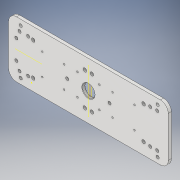
# Autodesk Inventor part: Base Plate New
Saved by Autodesk Inventor 2019 (Build 230136000, 136)
## iProperties
Created: 2019-10-06
Part Number: Base Plate New
Material: UHMW, White
Document SubType Name: Modeling
Designer: robgr
Density: 0.94 g/cm^3
Appearance: Smooth - White
Mass: 52.7671 g
Surface Area: 319.531 cm^2
Volume: 56.1352 cm^3
Author: robgr
Autodesk Inventor part; units mm, degrees
(part 1 of 2)
ref_plane "YZ Plane" through (0, 0, 0) normal (1, 0, 0) x (0, 1, 0)
sketch "Sketch1" plane through (0, 0, 0) normal (0, 0, 1) x (1, 0, 0)
  line L0 (-19.3782, 63.0791) -> (164.6218, 63.0791)
  line L1 (174.6218, 53.0791) -> (174.6218, 1.0791)
  line L2 (164.6218, -8.9209) -> (-19.3782, -8.9209)
  line L3 (-29.3782, 1.0791) -> (-29.3782, 53.0791)
  arc A0 (-19.3782, 63.0791) -> (-29.3782, 53.0791) centre (-19.3782, 53.0791) ccw
  arc A1 (-29.3782, 1.0791) -> (-19.3782, -8.9209) centre (-19.3782, 1.0791) ccw
  arc A2 (164.6218, -8.9209) -> (174.6218, 1.0791) centre (164.6218, 1.0791) ccw
  arc A3 (174.6218, 53.0791) -> (164.6218, 63.0791) centre (164.6218, 53.0791) ccw
  point P0 (0, 0)
  point P1 (-29.3782, 63.0791)
  point P2 (174.6218, -8.9209)
  point P3 (-29.3782, -8.9209)
  dimension "d0" = 204
  dimension "d1" = 72
  dimension "d2" = 10
  constraints: 8 end point, 8 point on circle, 8 tangent, 6 point on line, 4 centre point, 3 equal radius, 2 parallel, 1 horizontal, 1 perpendicular
  measures "d0" distance of point (174.622, -8.921) point (-29.378, -8.921)
  measures "d1" distance of point (-29.378, -8.921) point (-29.378, 63.079)
  measures "d2" radius of A0
extrude "Extrusion1" add sketch "Sketch1" along normal blind 4
sketch "Sketch3" plane through (0, 0, 0) normal (0, 0, -1) x (-1, 0, 0)
  circle A0 centre (19.3782, 39.5791) radius 2
  line L0 (29.3782, 1.0791) -> (29.3782, 53.0791) projected
  circle A1 centre (19.3782, 14.5791) radius 2
  circle A2 centre (19.3782, 53.0791) radius 2 projected
  circle A3 centre (19.3782, 1.0791) radius 2 projected
  line L1 (29.3782, 53.0791) -> (29.3782, 1.0791) projected
  line L2 (29.3782, 27.0791) -> (-174.6218, 27.0791)
  line L3 (-174.6218, 1.0791) -> (-174.6218, 53.0791) projected
  point P0 (0, 0)
  dimension "d10" = 4
  dimension "d15" = 25
  dimension "d16" = 12.5
  constraints: 2 centre point, 2 end point, 2 midpoint
  measures "d10" diameter of A0
  measures "d15" distance of A1.centre A0.centre
  measures "d16" distance from line of L2 A0.centre
extrude "Extrusion3" cut sketch "Sketch3" against normal blind 6 contours A0 | A1
sketch "Sketch4" plane through (0, 0, 4) normal (0, 0, 1) x (1, 0, 0)
  circle A0 centre (-4.3782, 5.0791) radius 2
  circle A1 centre (-19.3782, 14.5791) radius 2 projected
  circle A2 centre (-4.3782, 49.0791) radius 2
  circle A3 centre (-19.3782, 39.5791) radius 2 projected
  line L0 (164.6218, 63.0791) -> (-19.3782, 63.0791) projected
  line L1 (72.6218, 63.0791) -> (72.6218, -8.9209)
  line L2 (-19.3782, -8.9209) -> (164.6218, -8.9209) projected
  circle A4 centre (151.6218, 5.0791) radius 2
  circle A5 centre (151.6218, 49.0791) radius 2
  line L3 (174.6218, 1.0791) -> (174.6218, 53.0791) projected
  line L4 (-29.3782, 53.0791) -> (-29.3782, 1.0791) projected
  point P0 (0, 0)
  dimension "d17" = 4
  dimension "d19" = 4
  dimension "d37" = 23
  dimension "d38" = 14
  dimension "d39" = 14
  dimension "d40" = 23
  dimension "d41" = 25
  dimension "d42" = 14
  dimension "d43" = 25
  dimension "d44" = 14
  constraints: 4 centre point, 2 end point, 2 midpoint
  measures "d17" diameter of A0
  measures "d19" diameter of A2
  measures "d37" distance from line of L3 A4.centre
  measures "d38" distance from line of L2 A4.centre
  measures "d39" distance from line of L0 A5.centre
  measures "d40" distance from line of L3 A5.centre
  measures "d41" distance from line of L4 A2.centre
  measures "d42" distance from line of L0 A2.centre
  measures "d43" distance from line of L4 A0.centre
  measures "d44" distance from line of L2 A0.centre
extrude "Extrusion4" cut sketch "Sketch4" against normal blind 60 contours A0 | A2 | A4 | A5
ref_plane "Work Plane1" through (74.6218, 1.0791, 0) normal (1, 0, 0) x (0, 0, -1)
ref_plane "Work Plane2" through (-19.3782, 27.0791, 0) normal (0, -1, 0) x (1, 0, 0)
ref_plane "Work Plane3" through (-19.3782, 27.0791, 4) normal (0, 1, 0) x (1, 0, 0)
sketch "Sketch7" plane through (0, 0, 4) normal (0, 0, 1) x (1, 0, 0)
  point P0 (0, 0)
sketch "Sketch8" plane through (0, 0, 4) normal (0, 0, 1) x (1, 0, 0)
  circle A0 centre (-13.8782, -1.9209) radius 2
  line L0 (-19.3782, -8.9209) -> (164.6218, -8.9209) projected
  line L1 (-29.3782, 53.0791) -> (-29.3782, 1.0791) projected
  circle A1 centre (-13.8782, 56.0791) radius 2
  line L2 (164.6218, 63.0791) -> (-19.3782, 63.0791) projected
  circle A2 centre (161.1218, 56.0791) radius 2
  line L3 (174.6218, 1.0791) -> (174.6218, 53.0791) projected
  circle A3 centre (161.1218, -1.9209) radius 2
  point P0 (0, 0)
  dimension "d45" = 4
  dimension "d46" = 7
  dimension "d47" = 15.5
  dimension "d48" = 4
  dimension "d49" = 7
  dimension "d50" = 15.5
  dimension "d51" = 4
  dimension "d52" = 7
  dimension "d53" = 13.5
  constraints: 4 centre point
  measures "d45" diameter of A0
  measures "d46" distance from line of L0 A0.centre
  measures "d47" distance from line of L1 A0.centre
  measures "d48" diameter of A1
  measures "d49" distance from line of L2 A1.centre
  measures "d50" distance from line of L1 A1.centre
  measures "d51" diameter of A2
  measures "d52" distance from line of L2 A2.centre
  measures "d53" distance from line of L3 A2.centre
extrude "Extrusion6" cut sketch "Sketch8" against normal blind 10
sketch "Sketch9" plane through (0, 0, 4) normal (0, 0, 1) x (1, 0, 0)
  line L0 (-29.3782, 53.0791) -> (-29.3782, 1.0791) projected
  line L1 (-29.3782, 27.0791) -> (174.6218, 27.0791)
  line L2 (174.6218, 53.0791) -> (174.6218, 1.0791) projected
  line L3 (164.6218, 63.0791) -> (-19.3782, 63.0791) projected
  line L4 (72.6218, 63.0791) -> (72.6218, -8.9209)
  line L5 (164.6218, -8.9209) -> (-19.3782, -8.9209) projected
  circle A0 centre (72.6218, 27.0791) radius 8
  circle A1 centre (13.7163, 41.0791) radius 1
  circle A2 centre (41.7163, 41.0791) radius 1.0089
  circle A3 centre (41.7163, 13.0791) radius 1
  circle A4 centre (13.7163, 13.0791) radius 1
  circle A5 centre (77.0888, 48.0791) radius 2.225
  circle A6 centre (143.1888, 48.0791) radius 2.225
  circle A7 centre (143.1888, 6.0791) radius 2.225
  circle A8 centre (77.0888, 6.0791) radius 2.225
  point P0 (0, 0)
  dimension "d56" = 16
  dimension "d57" = 2
  dimension "d58" = 2
  dimension "d59" = 28
  dimension "d60" = 28
  dimension "d61" = 28
  dimension "d62" = 28
  dimension "d63" = 22
  dimension "d64" = 4.45
  dimension "d65" = 66.1
  dimension "d66" = 4.45
  dimension "d67" = 42
  dimension "d68" = 42
  dimension "d69" = 66.1
  dimension "d70" = 15
  dimension "d71" = 15
  dimension "d73" = 22
  constraints: 9 centre point, 5 midpoint, 4 end point
  measures "d56" diameter of A0
  measures "d57" diameter of A1
  measures "d58" diameter of A3
  measures "d59" distance of A2.centre A1.centre
  measures "d60" distance of A4.centre A1.centre
  measures "d61" distance of A3.centre A4.centre
  measures "d62" distance of A2.centre A3.centre
  measures "d63" distance from line of L3 A1.centre
  measures "d64" diameter of A5
  measures "d65" distance of A5.centre A6.centre
  measures "d66" diameter of A7
  measures "d67" distance of A7.centre A6.centre
  measures "d68" distance of A8.centre A5.centre
  measures "d69" distance of A7.centre A8.centre
  measures "d70" distance from line of L3 A5.centre
  measures "d71" distance from line of L5 A8.centre
  measures "d73" distance from line of L5 A4.centre
extrude "Extrusion7" cut sketch "Sketch9" against normal blind 10
ref_plane "Work Plane4" through (72.6218, 1.0791, 0) normal (1, 0, 0) x (0, 0, -1)
mirror "Mirror2" about plane through (72.6218, 1.0791, 0) normal (1, 0, 0) of "Extrusion7"
sketch "Sketch10" plane through (0, 0, 4) normal (0, 0, 1) x (1, 0, 0)
  line L0 (164.6218, 63.0791) -> (-19.3782, 63.0791) projected
  line L1 (72.6218, 63.0791) -> (72.6218, -8.9209)
  line L2 (-19.3782, -8.9209) -> (164.6218, -8.9209) projected
  line L3 (-29.3782, 53.0791) -> (-29.3782, 1.0791) projected
  line L4 (-29.3782, 27.0791) -> (174.6218, 27.0791)
  line L5 (174.6218, 1.0791) -> (174.6218, 53.0791) projected
  circle A0 centre (-15.3782, 49.0791) radius 2
  circle A1 centre (160.6218, 49.0791) radius 2
  circle A2 centre (-15.3782, 5.0791) radius 2
  circle A3 centre (160.6218, 5.0791) radius 2
  point P0 (0, 0)
  dimension "d77" = 4
  dimension "d78" = 14
  dimension "d79" = 14
  constraints: 4 centre point, 4 end point, 4 midpoint, 3 symmetric about line, 3 other
  measures "d77" diameter of A0
  measures "d78" distance from line of L0 A0.centre
  measures "d79" distance from line of L3 A0.centre
extrude "Extrusion8" cut sketch "Sketch10" against normal blind 10
sketch "Sketch11" plane through (0, 0, 4) normal (0, 0, 1) x (1, 0, 0)
  circle A0 centre (58.6218, 13.0791) radius 1.1
  circle A1 centre (58.6218, 41.0791) radius 1.1
  circle A2 centre (86.6218, 41.0791) radius 1.1
  circle A3 centre (86.6218, 13.0791) radius 1.1
  circle A4 centre (72.6218, 27.0791) radius 8 projected
  point P0 (0, 0)
  dimension "d82" = 2.2
  dimension "d83" = 2.2
  dimension "d84" = 2.2
  dimension "d85" = 28
  dimension "d86" = 28
  dimension "d87" = 28
  dimension "d88" = 28
  dimension "d89" = 14
  dimension "d90" = 14
  dimension "d91" = 14
  dimension "d92" = 14
  constraints: 4 centre point
  measures "d82" diameter of A0
  measures "d83" diameter of A1
  measures "d84" diameter of A2
  measures "d85" distance of A2.centre A1.centre
  measures "d86" distance of A1.centre A0.centre
  measures "d87" distance of A3.centre A0.centre
  measures "d88" distance of A2.centre A3.centre
  measures "d89" horizontal distance of A0.centre A4.centre
  measures "d90" horizontal distance of A3.centre A4.centre
  measures "d91" horizontal distance of A2.centre A4.centre
  measures "d92" horizontal distance of A4.centre A1.centre
extrude "Extrusion9" cut sketch "Sketch11" against normal blind 10 contours A0 | A1 | A2 | A3
fillet "Fillet1" radius 0.5 2 edges at (64.6218, 27.0791, 4) (64.6218, 27.0791, 0)
sketch "Sketch12" plane through (0, 0, 4) normal (0, 0, 1) x (1, 0, 0)
  line L0 (-29.3782, 1.0791) -> (-29.3782, 53.0791) projected
  line L1 (-29.3782, 27.0791) -> (174.6218, 27.0791)
  line L2 (174.6218, 53.0791) -> (174.6218, 1.0791) projected
  circle A0 centre (45.6218, 27.0791) radius 2
  circle A1 centre (99.6218, 27.0791) radius 2
  point P0 (0, 0)
  dimension "d96" = 4
  dimension "d97" = 4
  dimension "d98" = 75
  dimension "d99" = 75
  constraints: 2 centre point, 2 end point, 2 midpoint, 2 point on line
  measures "d96" diameter of A0
  measures "d97" diameter of A1
  measures "d98" distance from line of L0 A0.centre
  measures "d99" distance from line of L2 A1.centre
extrude "Extrusion10" cut sketch "Sketch12" against normal blind 10
sketch "Sketch13" plane through (0, 0, 0) normal (0, 0, -1) x (-1, 0, 0)
  line L0 (-128.4589, -1.8253) -> (-20.3883, -1.8253) construction
  line L1 (-20.3883, -1.8253) -> (-20.3883, -5.9209) construction
  line L2 (-20.3883, -5.9209) -> (-128.4589, -5.9209) construction
  line L3 (-128.4589, -5.9209) -> (-128.4589, -1.8253) construction
  line L4 (-164.6218, -8.9209) -> (19.3782, -8.9209) projected
  line L5 (-60.6379, 54.6498) -> (-88.5532, 54.6498) construction
  line L6 (-88.5532, 54.6498) -> (-88.5532, 60.0791) construction
  line L7 (-88.5532, 60.0791) -> (-60.6379, 60.0791) construction
  line L8 (-60.6379, 60.0791) -> (-60.6379, 54.6498) construction
  line L9 (19.3782, 63.0791) -> (-164.6218, 63.0791) projected
  line L10 (-125.7913, -5.029) -> (-126.3174, -5.029)
  line L11 (-126.3174, -5.029) -> (-127.2807, -3.8162)
  line L12 (-127.2807, -3.8162) -> (-127.7451, -3.8162)
  line L13 (-127.7451, -3.8162) -> (-127.7451, -5.029)
  line L14 (-127.7451, -5.029) -> (-128.1501, -5.029)
  line L15 (-128.1501, -5.029) -> (-128.1501, -1.981)
  line L16 (-128.1501, -1.981) -> (-127.3647, -1.981)
  spline S0 degree 2 poles (-127.3647, -1.981) (-127.1029, -1.981) (-126.7496, -2.0378) (-126.5891, -2.1415) knots 0 0 0 1 2 2 2
  spline S1 degree 2 poles (-126.5891, -2.1415) (-126.4285, -2.2452) (-126.2433, -2.5688) (-126.2433, -2.8084) knots 0 0 0 1 2 2 2
  spline S2 degree 2 poles (-126.2433, -2.8084) (-126.2433, -3.1419) (-126.5841, -3.5939) (-126.8756, -3.7026) knots 0 0 0 1 2 2 2
  line L17 (-126.8756, -3.7026) -> (-125.7913, -5.029)
  spline S3 degree 2 poles (-126.6657, -2.8405) (-126.6657, -2.7071) (-126.7595, -2.5021) (-126.8583, -2.4354) knots 0 0 0 1 2 2 2
  spline S4 degree 2 poles (-126.8583, -2.4354) (-126.9448, -2.3786) (-127.1745, -2.3317) (-127.3424, -2.3317) knots 0 0 0 1 2 2 2
  line L18 (-127.3424, -2.3317) -> (-127.7451, -2.3317)
  line L19 (-127.7451, -2.3317) -> (-127.7451, -3.4778)
  line L20 (-127.7451, -3.4778) -> (-127.3894, -3.4778)
  spline S5 degree 2 poles (-127.3894, -3.4778) (-127.214, -3.4778) (-126.9349, -3.416) (-126.8386, -3.3197) knots 0 0 0 1 2 2 2
  spline S6 degree 2 poles (-126.8386, -3.3197) (-126.7496, -3.2357) (-126.6657, -2.9986) (-126.6657, -2.8405) knots 0 0 0 1 2 2 2
  spline S7 degree 2 poles (-123.6992, -3.8853) (-123.6992, -4.4633) (-124.2549, -5.0932) (-124.7193, -5.0932) knots 0 0 0 1 2 2 2
  spline S8 degree 2 poles (-124.7193, -5.0932) (-125.196, -5.0932) (-125.7419, -4.4436) (-125.7419, -3.8853) knots 0 0 0 1 2 2 2
  spline S9 degree 2 poles (-125.7419, -3.8853) (-125.7419, -3.3123) (-125.1787, -2.6775) (-124.7193, -2.6775) knots 0 0 0 1 2 2 2
  spline S10 degree 2 poles (-124.7193, -2.6775) (-124.2549, -2.6775) (-123.6992, -3.3098) (-123.6992, -3.8853) knots 0 0 0 1 2 2 2
  spline S11 degree 2 poles (-124.0968, -3.8853) (-124.0968, -3.4407) (-124.4204, -3.0085) (-124.7193, -3.0085) knots 0 0 0 1 2 2 2
  spline S12 degree 2 poles (-124.7193, -3.0085) (-125.0182, -3.0085) (-125.3442, -3.4407) (-125.3442, -3.8853) knots 0 0 0 1 2 2 2
  spline S13 degree 2 poles (-125.3442, -3.8853) (-125.3442, -4.3176) (-125.0182, -4.7622) (-124.7193, -4.7622) knots 0 0 0 1 2 2 2
  spline S14 degree 2 poles (-124.7193, -4.7622) (-124.4229, -4.7622) (-124.0968, -4.325) (-124.0968, -3.8853) knots 0 0 0 1 2 2 2
  spline S15 degree 2 poles (-121.3872, -3.8483) (-121.3872, -4.409) (-121.9306, -5.0932) (-122.3407, -5.0932) knots 0 0 0 1 2 2 2
  spline S16 degree 2 poles (-122.3407, -5.0932) (-122.5259, -5.0932) (-122.7902, -5.0018) (-122.9186, -4.9227) knots 0 0 0 1 2 2 2
  line L21 (-122.9186, -4.9227) -> (-122.9433, -5.029)
  line L22 (-122.9433, -5.029) -> (-123.304, -5.029)
  line L23 (-123.304, -5.029) -> (-123.304, -1.8451)
  line L24 (-123.304, -1.8451) -> (-122.9186, -1.8451)
  line L25 (-122.9186, -1.8451) -> (-122.9186, -2.9813)
  spline S17 degree 2 poles (-122.9186, -2.9813) (-122.7729, -2.8504) (-122.4345, -2.6775) (-122.2196, -2.6775) knots 0 0 0 1 2 2 2
  spline S18 degree 2 poles (-122.2196, -2.6775) (-121.8318, -2.6775) (-121.3872, -3.2975) (-121.3872, -3.8483) knots 0 0 0 1 2 2 2
  spline S19 degree 2 poles (-121.7849, -3.8779) (-121.7849, -3.4679) (-122.0344, -3.0431) (-122.311, -3.0431) knots 0 0 0 1 2 2 2
  spline S20 degree 2 poles (-122.311, -3.0431) (-122.4666, -3.0431) (-122.7877, -3.1913) (-122.9186, -3.3049) knots 0 0 0 1 2 2 2
  line L26 (-122.9186, -3.3049) -> (-122.9186, -4.6165)
  spline S21 degree 2 poles (-122.9186, -4.6165) (-122.7729, -4.6881) (-122.5481, -4.7474) (-122.4148, -4.7474) knots 0 0 0 1 2 2 2
  spline S22 degree 2 poles (-122.4148, -4.7474) (-122.1208, -4.7474) (-121.7849, -4.3299) (-121.7849, -3.8779) knots 0 0 0 1 2 2 2
  spline S23 degree 2 poles (-118.3713, -5.0882) (-118.6949, -5.0882) (-119.2309, -4.8906) (-119.4236, -4.6906) knots 0 0 0 1 2 2 2
  spline S24 degree 2 poles (-119.4236, -4.6906) (-119.6162, -4.488) (-119.8212, -3.8903) (-119.8212, -3.5025) knots 0 0 0 1 2 2 2
  spline S25 degree 2 poles (-119.8212, -3.5025) (-119.8212, -3.1344) (-119.6138, -2.5515) (-119.4211, -2.344) knots 0 0 0 1 2 2 2
  spline S26 degree 2 poles (-119.4211, -2.344) (-119.2359, -2.144) (-118.6924, -1.9266) (-118.3689, -1.9266) knots 0 0 0 1 2 2 2
  spline S27 degree 2 poles (-118.3689, -1.9266) (-118.2133, -1.9266) (-117.9317, -1.9711) (-117.8032, -2.0106) knots 0 0 0 1 2 2 2
  spline S28 degree 2 poles (-117.8032, -2.0106) (-117.6995, -2.0402) (-117.4476, -2.1489) (-117.371, -2.1884) knots 0 0 0 1 2 2 2
  line L27 (-117.371, -2.1884) -> (-117.371, -2.6775)
  line L28 (-117.371, -2.6775) -> (-117.4056, -2.6775)
  spline S29 degree 2 poles (-117.4056, -2.6775) (-117.4821, -2.6108) (-117.6427, -2.4898) (-117.7909, -2.4206) knots 0 0 0 1 2 2 2
  spline S30 degree 2 poles (-117.7909, -2.4206) (-117.9144, -2.3589) (-118.233, -2.2774) (-118.4158, -2.2774) knots 0 0 0 1 2 2 2
  spline S31 degree 2 poles (-118.4158, -2.2774) (-118.8555, -2.2774) (-119.3989, -2.9393) (-119.3989, -3.4901) knots 0 0 0 1 2 2 2
  spline S32 degree 2 poles (-119.3989, -3.4901) (-119.3989, -3.7964) (-119.2556, -4.2558) (-119.1198, -4.4139) knots 0 0 0 1 2 2 2
  spline S33 degree 2 poles (-119.1198, -4.4139) (-118.9888, -4.572) (-118.6183, -4.7375) (-118.3862, -4.7375) knots 0 0 0 1 2 2 2
  spline S34 degree 2 poles (-118.3862, -4.7375) (-118.2157, -4.7375) (-117.8749, -4.6881) (-117.7588, -4.6387) knots 0 0 0 1 2 2 2
  line L29 (-117.7588, -4.6387) -> (-117.7588, -3.8508)
  line L30 (-117.7588, -3.8508) -> (-118.4652, -3.8508)
  line L31 (-118.4652, -3.8508) -> (-118.4652, -3.4951)
  line L32 (-118.4652, -3.4951) -> (-117.3586, -3.4951)
  line L33 (-117.3586, -3.4951) -> (-117.3586, -4.8264)
  spline S35 degree 2 poles (-117.3586, -4.8264) (-117.4352, -4.861) (-117.697, -4.9672) (-117.8082, -4.9993) knots 0 0 0 1 2 2 2
  spline S36 degree 2 poles (-117.8082, -4.9993) (-117.9589, -5.0438) (-118.2009, -5.0882) (-118.3713, -5.0882) knots 0 0 0 1 2 2 2
  line L34 (-115.6667, -3.1542) -> (-115.6864, -3.1542)
  spline S37 degree 2 poles (-115.6864, -3.1542) (-115.7309, -3.1419) (-115.8272, -3.1369) (-115.8939, -3.1369) knots 0 0 0 1 2 2 2
  spline S38 degree 2 poles (-115.8939, -3.1369) (-116.0495, -3.1369) (-116.3558, -3.2728) (-116.4941, -3.4062) knots 0 0 0 1 2 2 2
  line L35 (-116.4941, -3.4062) -> (-116.4941, -5.029)
  line L36 (-116.4941, -5.029) -> (-116.8795, -5.029)
  line L37 (-116.8795, -5.029) -> (-116.8795, -2.7417)
  line L38 (-116.8795, -2.7417) -> (-116.4941, -2.7417)
  line L39 (-116.4941, -2.7417) -> (-116.4941, -3.0826)
  spline S39 degree 2 poles (-116.4941, -3.0826) (-116.2842, -2.8949) (-115.9705, -2.7417) (-115.8223, -2.7417) knots 0 0 0 1 2 2 2
  spline S40 degree 2 poles (-115.8223, -2.7417) (-115.763, -2.7417) (-115.7037, -2.7467) (-115.6667, -2.7541) knots 0 0 0 1 2 2 2
  line L40 (-115.6667, -2.7541) -> (-115.6667, -3.1542)
  line L41 (-113.5894, -5.029) -> (-113.9747, -5.029)
  line L42 (-113.9747, -5.029) -> (-113.9747, -4.777)
  spline S41 degree 2 poles (-113.9747, -4.777) (-114.1526, -4.9326) (-114.4712, -5.0932) (-114.6688, -5.0932) knots 0 0 0 1 2 2 2
  spline S42 degree 2 poles (-114.6688, -5.0932) (-114.817, -5.0932) (-115.0813, -4.9944) (-115.1776, -4.8882) knots 0 0 0 1 2 2 2
  spline S43 degree 2 poles (-115.1776, -4.8882) (-115.2764, -4.782) (-115.3851, -4.4584) (-115.3851, -4.2262) knots 0 0 0 1 2 2 2
  line L43 (-115.3851, -4.2262) -> (-115.3851, -2.7417)
  line L44 (-115.3851, -2.7417) -> (-114.9998, -2.7417)
  line L45 (-114.9998, -2.7417) -> (-114.9998, -4.0459)
  spline S44 degree 2 poles (-114.9998, -4.0459) (-114.9998, -4.2287) (-114.9726, -4.4683) (-114.9257, -4.5572) knots 0 0 0 1 2 2 2
  spline S45 degree 2 poles (-114.9257, -4.5572) (-114.8787, -4.6461) (-114.7182, -4.7276) (-114.5675, -4.7276) knots 0 0 0 1 2 2 2
  spline S46 degree 2 poles (-114.5675, -4.7276) (-114.4267, -4.7276) (-114.1081, -4.5671) (-113.9747, -4.451) knots 0 0 0 1 2 2 2
  line L46 (-113.9747, -4.451) -> (-113.9747, -2.7417)
  line L47 (-113.9747, -2.7417) -> (-113.5894, -2.7417)
  line L48 (-113.5894, -2.7417) -> (-113.5894, -5.029)
  spline S47 degree 2 poles (-112.4137, -5.0833) (-112.6434, -5.0833) (-113.0411, -4.9598) (-113.172, -4.8906) knots 0 0 0 1 2 2 2
  line L49 (-113.172, -4.8906) -> (-113.172, -4.4584)
  line L50 (-113.172, -4.4584) -> (-113.1522, -4.4584)
  spline S48 degree 2 poles (-113.1522, -4.4584) (-113.1028, -4.4979) (-112.9694, -4.5918) (-112.8583, -4.6436) knots 0 0 0 1 2 2 2
  spline S49 degree 2 poles (-112.8583, -4.6436) (-112.7619, -4.6906) (-112.5248, -4.7597) (-112.3988, -4.7597) knots 0 0 0 1 2 2 2
  spline S50 degree 2 poles (-112.3988, -4.7597) (-112.3075, -4.7597) (-112.0975, -4.7177) (-112.0481, -4.6831) knots 0 0 0 1 2 2 2
  spline S51 degree 2 poles (-112.0481, -4.6831) (-111.9765, -4.6362) (-111.9123, -4.53) (-111.9123, -4.4213) knots 0 0 0 1 2 2 2
  spline S52 degree 2 poles (-111.9123, -4.4213) (-111.9123, -4.2855) (-112.0605, -4.1447) (-112.2506, -4.0978) knots 0 0 0 1 2 2 2
  spline S53 degree 2 poles (-112.2506, -4.0978) (-112.3247, -4.0805) (-112.5619, -4.0311) (-112.6631, -4.0039) knots 0 0 0 1 2 2 2
  spline S54 degree 2 poles (-112.6631, -4.0039) (-112.925, -3.9273) (-113.1621, -3.6112) (-113.1621, -3.3864) knots 0 0 0 1 2 2 2
  spline S55 degree 2 poles (-113.1621, -3.3864) (-113.1621, -3.0752) (-112.6952, -2.6874) (-112.3099, -2.6874) knots 0 0 0 1 2 2 2
  spline S56 degree 2 poles (-112.3099, -2.6874) (-112.1197, -2.6874) (-111.7344, -2.7812) (-111.6035, -2.8529) knots 0 0 0 1 2 2 2
  line L51 (-111.6035, -2.8529) -> (-111.6035, -3.2654)
  line L52 (-111.6035, -3.2654) -> (-111.6233, -3.2654)
  spline S57 degree 2 poles (-111.6233, -3.2654) (-111.7715, -3.1468) (-112.1321, -3.0109) (-112.3173, -3.0109) knots 0 0 0 1 2 2 2
  spline S58 degree 2 poles (-112.3173, -3.0109) (-112.5075, -3.0109) (-112.7693, -3.1715) (-112.7693, -3.3321) knots 0 0 0 1 2 2 2
  spline S59 degree 2 poles (-112.7693, -3.3321) (-112.7693, -3.4778) (-112.6137, -3.6186) (-112.4408, -3.663) knots 0 0 0 1 2 2 2
  spline S60 degree 2 poles (-112.4408, -3.663) (-112.3569, -3.6853) (-112.1444, -3.7297) (-112.0283, -3.7569) knots 0 0 0 1 2 2 2
  spline S61 degree 2 poles (-112.0283, -3.7569) (-111.7764, -3.8211) (-111.5195, -4.115) (-111.5195, -4.3695) knots 0 0 0 1 2 2 2
  spline S62 degree 2 poles (-111.5195, -4.3695) (-111.5195, -4.5177) (-111.6356, -4.7795) (-111.7492, -4.8758) knots 0 0 0 1 2 2 2
  spline S63 degree 2 poles (-111.7492, -4.8758) (-111.8703, -4.9771) (-112.179, -5.0833) (-112.4137, -5.0833) knots 0 0 0 1 2 2 2
  line L53 (-109.2669, -5.029) -> (-109.7732, -5.029)
  line L54 (-109.7732, -5.029) -> (-110.6229, -3.9249)
  line L55 (-110.6229, -3.9249) -> (-110.776, -4.0731)
  line L56 (-110.776, -4.0731) -> (-110.776, -5.029)
  line L57 (-110.776, -5.029) -> (-111.1614, -5.029)
  line L58 (-111.1614, -5.029) -> (-111.1614, -1.8451)
  line L59 (-111.1614, -1.8451) -> (-110.776, -1.8451)
  line L60 (-110.776, -1.8451) -> (-110.776, -3.7075)
  line L61 (-110.776, -3.7075) -> (-109.872, -2.7417)
  line L62 (-109.872, -2.7417) -> (-109.3928, -2.7417)
  line L63 (-109.3928, -2.7417) -> (-110.3314, -3.6976)
  line L64 (-110.3314, -3.6976) -> (-109.2669, -5.029)
  line L65 (-108.6815, -5.029) -> (-109.0668, -5.029)
  line L66 (-109.0668, -5.029) -> (-109.0668, -2.7417)
  line L67 (-109.0668, -2.7417) -> (-108.6815, -2.7417)
  line L68 (-108.6815, -2.7417) -> (-108.6815, -5.029)
  line L69 (-108.6543, -2.3613) -> (-109.0915, -2.3613)
  line L70 (-109.0915, -2.3613) -> (-109.0915, -1.9612)
  line L71 (-109.0915, -1.9612) -> (-108.6543, -1.9612)
  line L72 (-108.6543, -1.9612) -> (-108.6543, -2.3613)
  line L73 (-106.3201, -5.029) -> (-106.7055, -5.029)
  line L74 (-106.7055, -5.029) -> (-106.7055, -3.7248)
  spline S64 degree 2 poles (-106.7055, -3.7248) (-106.7055, -3.5667) (-106.7351, -3.295) (-106.7796, -3.2135) knots 0 0 0 1 2 2 2
  spline S65 degree 2 poles (-106.7796, -3.2135) (-106.8265, -3.127) (-106.9945, -3.0431) (-107.1377, -3.0431) knots 0 0 0 1 2 2 2
  spline S66 degree 2 poles (-107.1377, -3.0431) (-107.281, -3.0431) (-107.5848, -3.1962) (-107.7305, -3.3197) knots 0 0 0 1 2 2 2
  line L75 (-107.7305, -3.3197) -> (-107.7305, -5.029)
  line L76 (-107.7305, -5.029) -> (-108.1158, -5.029)
  line L77 (-108.1158, -5.029) -> (-108.1158, -2.7417)
  line L78 (-108.1158, -2.7417) -> (-107.7305, -2.7417)
  line L79 (-107.7305, -2.7417) -> (-107.7305, -2.9961)
  spline S67 degree 2 poles (-107.7305, -2.9961) (-107.5576, -2.8405) (-107.2242, -2.6775) (-107.0364, -2.6775) knots 0 0 0 1 2 2 2
  spline S68 degree 2 poles (-107.0364, -2.6775) (-106.7005, -2.6775) (-106.3201, -3.1221) (-106.3201, -3.5445) knots 0 0 0 1 2 2 2
  line L80 (-106.3201, -3.5445) -> (-106.3201, -5.029)
  line L81 (-103.4105, -3.8804) -> (-104.564, -3.8804)
  line L82 (-104.564, -3.8804) -> (-104.564, -3.5099)
  line L83 (-104.564, -3.5099) -> (-103.4105, -3.5099)
  line L84 (-103.4105, -3.5099) -> (-103.4105, -3.8804)
  spline S69 degree 2 poles (-100.3328, -5.0882) (-100.6564, -5.0882) (-101.1924, -4.8906) (-101.385, -4.6906) knots 0 0 0 1 2 2 2
  spline S70 degree 2 poles (-101.385, -4.6906) (-101.5777, -4.488) (-101.7827, -3.8903) (-101.7827, -3.5025) knots 0 0 0 1 2 2 2
  spline S71 degree 2 poles (-101.7827, -3.5025) (-101.7827, -3.1344) (-101.5752, -2.5515) (-101.3826, -2.344) knots 0 0 0 1 2 2 2
  spline S72 degree 2 poles (-101.3826, -2.344) (-101.1973, -2.144) (-100.6539, -1.9266) (-100.3303, -1.9266) knots 0 0 0 1 2 2 2
  spline S73 degree 2 poles (-100.3303, -1.9266) (-100.1747, -1.9266) (-99.8932, -1.9711) (-99.7647, -2.0106) knots 0 0 0 1 2 2 2
  spline S74 degree 2 poles (-99.7647, -2.0106) (-99.661, -2.0402) (-99.409, -2.1489) (-99.3325, -2.1884) knots 0 0 0 1 2 2 2
  line L85 (-99.3325, -2.1884) -> (-99.3325, -2.6775)
  line L86 (-99.3325, -2.6775) -> (-99.367, -2.6775)
  spline S75 degree 2 poles (-99.367, -2.6775) (-99.4436, -2.6108) (-99.6042, -2.4898) (-99.7524, -2.4206) knots 0 0 0 1 2 2 2
  spline S76 degree 2 poles (-99.7524, -2.4206) (-99.8759, -2.3589) (-100.1945, -2.2774) (-100.3773, -2.2774) knots 0 0 0 1 2 2 2
  spline S77 degree 2 poles (-100.3773, -2.2774) (-100.8169, -2.2774) (-101.3603, -2.9393) (-101.3603, -3.4901) knots 0 0 0 1 2 2 2
  spline S78 degree 2 poles (-101.3603, -3.4901) (-101.3603, -3.7964) (-101.2171, -4.2558) (-101.0812, -4.4139) knots 0 0 0 1 2 2 2
  spline S79 degree 2 poles (-101.0812, -4.4139) (-100.9503, -4.572) (-100.5798, -4.7375) (-100.3476, -4.7375) knots 0 0 0 1 2 2 2
  spline S80 degree 2 poles (-100.3476, -4.7375) (-100.1772, -4.7375) (-99.8363, -4.6881) (-99.7203, -4.6387) knots 0 0 0 1 2 2 2
  line L87 (-99.7203, -4.6387) -> (-99.7203, -3.8508)
  line L88 (-99.7203, -3.8508) -> (-100.4267, -3.8508)
  line L89 (-100.4267, -3.8508) -> (-100.4267, -3.4951)
  line L90 (-100.4267, -3.4951) -> (-99.3201, -3.4951)
  line L91 (-99.3201, -3.4951) -> (-99.3201, -4.8264)
  spline S81 degree 2 poles (-99.3201, -4.8264) (-99.3967, -4.861) (-99.6585, -4.9672) (-99.7697, -4.9993) knots 0 0 0 1 2 2 2
  spline S82 degree 2 poles (-99.7697, -4.9993) (-99.9203, -5.0438) (-100.1624, -5.0882) (-100.3328, -5.0882) knots 0 0 0 1 2 2 2
  spline S83 degree 2 poles (-97.848, -5.0808) (-98.3963, -5.0808) (-98.999, -4.4658) (-98.999, -3.8977) knots 0 0 0 1 2 2 2
  spline S84 degree 2 poles (-98.999, -3.8977) (-98.999, -3.3395) (-98.4136, -2.6775) (-97.9418, -2.6775) knots 0 0 0 1 2 2 2
  spline S85 degree 2 poles (-97.9418, -2.6775) (-97.7294, -2.6775) (-97.4009, -2.801) (-97.2799, -2.9319) knots 0 0 0 1 2 2 2
  spline S86 degree 2 poles (-97.2799, -2.9319) (-97.1564, -3.0628) (-97.0255, -3.4407) (-97.0255, -3.7149) knots 0 0 0 1 2 2 2
  line L92 (-97.0255, -3.7149) -> (-97.0255, -3.9249)
  line L93 (-97.0255, -3.9249) -> (-98.6087, -3.9249)
  spline S87 degree 2 poles (-98.6087, -3.9249) (-98.6087, -4.3225) (-98.2086, -4.7449) (-97.8529, -4.7449) knots 0 0 0 1 2 2 2
  spline S88 degree 2 poles (-97.8529, -4.7449) (-97.7269, -4.7449) (-97.4824, -4.6881) (-97.3836, -4.6436) knots 0 0 0 1 2 2 2
  spline S89 degree 2 poles (-97.3836, -4.6436) (-97.2799, -4.5942) (-97.1366, -4.5078) (-97.0897, -4.4683) knots 0 0 0 1 2 2 2
  line L94 (-97.0897, -4.4683) -> (-97.0675, -4.4683)
  line L95 (-97.0675, -4.4683) -> (-97.0675, -4.8882)
  spline S90 degree 2 poles (-97.0675, -4.8882) (-97.1341, -4.9153) (-97.3367, -4.9944) (-97.4157, -5.0166) knots 0 0 0 1 2 2 2
  spline S91 degree 2 poles (-97.4157, -5.0166) (-97.5269, -5.0487) (-97.7097, -5.0808) (-97.848, -5.0808) knots 0 0 0 1 2 2 2
  spline S92 degree 2 poles (-97.4009, -3.6309) (-97.4058, -3.4753) (-97.4701, -3.2481) (-97.5318, -3.1715) knots 0 0 0 1 2 2 2
  spline S93 degree 2 poles (-97.5318, -3.1715) (-97.5985, -3.085) (-97.8085, -2.9937) (-97.9641, -2.9937) knots 0 0 0 1 2 2 2
  spline S94 degree 2 poles (-97.9641, -2.9937) (-98.1172, -2.9937) (-98.3321, -3.085) (-98.421, -3.174) knots 0 0 0 1 2 2 2
  spline S95 degree 2 poles (-98.421, -3.174) (-98.5075, -3.2654) (-98.5964, -3.4852) (-98.6087, -3.6309) knots 0 0 0 1 2 2 2
  line L96 (-98.6087, -3.6309) -> (-97.4009, -3.6309)
  spline S96 degree 2 poles (-94.7555, -3.8853) (-94.7555, -4.4633) (-95.3113, -5.0932) (-95.7756, -5.0932) knots 0 0 0 1 2 2 2
  spline S97 degree 2 poles (-95.7756, -5.0932) (-96.2524, -5.0932) (-96.7982, -4.4436) (-96.7982, -3.8853) knots 0 0 0 1 2 2 2
  spline S98 degree 2 poles (-96.7982, -3.8853) (-96.7982, -3.3123) (-96.2351, -2.6775) (-95.7756, -2.6775) knots 0 0 0 1 2 2 2
  spline S99 degree 2 poles (-95.7756, -2.6775) (-95.3113, -2.6775) (-94.7555, -3.3098) (-94.7555, -3.8853) knots 0 0 0 1 2 2 2
  spline S100 degree 2 poles (-95.1532, -3.8853) (-95.1532, -3.4407) (-95.4768, -3.0085) (-95.7756, -3.0085) knots 0 0 0 1 2 2 2
  spline S101 degree 2 poles (-95.7756, -3.0085) (-96.0745, -3.0085) (-96.4006, -3.4407) (-96.4006, -3.8853) knots 0 0 0 1 2 2 2
  spline S102 degree 2 poles (-96.4006, -3.8853) (-96.4006, -4.3176) (-96.0745, -4.7622) (-95.7756, -4.7622) knots 0 0 0 1 2 2 2
  spline S103 degree 2 poles (-95.7756, -4.7622) (-95.4792, -4.7622) (-95.1532, -4.325) (-95.1532, -3.8853) knots 0 0 0 1 2 2 2
  line L97 (-93.1475, -3.1542) -> (-93.1673, -3.1542)
  spline S104 degree 2 poles (-93.1673, -3.1542) (-93.2118, -3.1419) (-93.3081, -3.1369) (-93.3748, -3.1369) knots 0 0 0 1 2 2 2
  spline S105 degree 2 poles (-93.3748, -3.1369) (-93.5304, -3.1369) (-93.8367, -3.2728) (-93.975, -3.4062) knots 0 0 0 1 2 2 2
  line L98 (-93.975, -3.4062) -> (-93.975, -5.029)
  line L99 (-93.975, -5.029) -> (-94.3603, -5.029)
  line L100 (-94.3603, -5.029) -> (-94.3603, -2.7417)
  line L101 (-94.3603, -2.7417) -> (-93.975, -2.7417)
  line L102 (-93.975, -2.7417) -> (-93.975, -3.0826)
  spline S106 degree 2 poles (-93.975, -3.0826) (-93.765, -2.8949) (-93.4514, -2.7417) (-93.3032, -2.7417) knots 0 0 0 1 2 2 2
  spline S107 degree 2 poles (-93.3032, -2.7417) (-93.2439, -2.7417) (-93.1846, -2.7467) (-93.1475, -2.7541) knots 0 0 0 1 2 2 2
  line L103 (-93.1475, -2.7541) -> (-93.1475, -3.1542)
  line L104 (-91.09, -5.029) -> (-91.4753, -5.029)
  line L105 (-91.4753, -5.029) -> (-91.4753, -4.7968)
  spline S108 degree 2 poles (-91.4753, -4.7968) (-91.5643, -4.8709) (-91.6952, -4.9697) (-91.7841, -5.0117) knots 0 0 0 1 2 2 2
  spline S109 degree 2 poles (-91.7841, -5.0117) (-91.8656, -5.0512) (-92.041, -5.0932) (-92.1571, -5.0932) knots 0 0 0 1 2 2 2
  spline S110 degree 2 poles (-92.1571, -5.0932) (-92.3448, -5.0932) (-92.6609, -4.9376) (-92.7721, -4.7869) knots 0 0 0 1 2 2 2
  spline S111 degree 2 poles (-92.7721, -4.7869) (-92.8832, -4.6362) (-93.0067, -4.1916) (-93.0067, -3.9026) knots 0 0 0 1 2 2 2
  spline S112 degree 2 poles (-93.0067, -3.9026) (-93.0067, -3.6013) (-92.8511, -3.1616) (-92.7153, -2.9961) knots 0 0 0 1 2 2 2
  spline S113 degree 2 poles (-92.7153, -2.9961) (-92.5893, -2.8479) (-92.2361, -2.6775) (-92.041, -2.6775) knots 0 0 0 1 2 2 2
  spline S114 degree 2 poles (-92.041, -2.6775) (-91.8705, -2.6775) (-91.6161, -2.7541) (-91.4753, -2.8331) knots 0 0 0 1 2 2 2
  line L106 (-91.4753, -2.8331) -> (-91.4753, -1.8451)
  line L107 (-91.4753, -1.8451) -> (-91.09, -1.8451)
  line L108 (-91.09, -1.8451) -> (-91.09, -5.029)
  line L109 (-91.4753, -4.4732) -> (-91.4753, -3.1517)
  spline S115 degree 2 poles (-91.4753, -3.1517) (-91.6186, -3.0826) (-91.8458, -3.0307) (-91.9768, -3.0307) knots 0 0 0 1 2 2 2
  spline S116 degree 2 poles (-91.9768, -3.0307) (-92.2732, -3.0307) (-92.6091, -3.4753) (-92.6091, -3.8952) knots 0 0 0 1 2 2 2
  spline S117 degree 2 poles (-92.6091, -3.8952) (-92.6091, -4.3003) (-92.3522, -4.7276) (-92.0681, -4.7276) knots 0 0 0 1 2 2 2
  spline S118 degree 2 poles (-92.0681, -4.7276) (-91.9175, -4.7276) (-91.6112, -4.5893) (-91.4753, -4.4732) knots 0 0 0 1 2 2 2
  line L110 (-90.1391, -5.029) -> (-90.5244, -5.029)
  line L111 (-90.5244, -5.029) -> (-90.5244, -2.7417)
  line L112 (-90.5244, -2.7417) -> (-90.1391, -2.7417)
  line L113 (-90.1391, -2.7417) -> (-90.1391, -5.029)
  line L114 (-90.1119, -2.3613) -> (-90.5491, -2.3613)
  line L115 (-90.5491, -2.3613) -> (-90.5491, -1.9612)
  line L116 (-90.5491, -1.9612) -> (-90.1119, -1.9612)
  line L117 (-90.1119, -1.9612) -> (-90.1119, -2.3613)
  spline S119 degree 2 poles (-88.5805, -5.0808) (-89.1288, -5.0808) (-89.7315, -4.4658) (-89.7315, -3.8977) knots 0 0 0 1 2 2 2
  spline S120 degree 2 poles (-89.7315, -3.8977) (-89.7315, -3.3395) (-89.1461, -2.6775) (-88.6743, -2.6775) knots 0 0 0 1 2 2 2
  spline S121 degree 2 poles (-88.6743, -2.6775) (-88.4619, -2.6775) (-88.1334, -2.801) (-88.0124, -2.9319) knots 0 0 0 1 2 2 2
  spline S122 degree 2 poles (-88.0124, -2.9319) (-87.8889, -3.0628) (-87.758, -3.4407) (-87.758, -3.7149) knots 0 0 0 1 2 2 2
  line L118 (-87.758, -3.7149) -> (-87.758, -3.9249)
  line L119 (-87.758, -3.9249) -> (-89.3412, -3.9249)
  spline S123 degree 2 poles (-89.3412, -3.9249) (-89.3412, -4.3225) (-88.9411, -4.7449) (-88.5854, -4.7449) knots 0 0 0 1 2 2 2
  spline S124 degree 2 poles (-88.5854, -4.7449) (-88.4594, -4.7449) (-88.2149, -4.6881) (-88.1161, -4.6436) knots 0 0 0 1 2 2 2
  spline S125 degree 2 poles (-88.1161, -4.6436) (-88.0124, -4.5942) (-87.8691, -4.5078) (-87.8222, -4.4683) knots 0 0 0 1 2 2 2
  line L120 (-87.8222, -4.4683) -> (-87.8, -4.4683)
  line L121 (-87.8, -4.4683) -> (-87.8, -4.8882)
  spline S126 degree 2 poles (-87.8, -4.8882) (-87.8666, -4.9153) (-88.0692, -4.9944) (-88.1482, -5.0166) knots 0 0 0 1 2 2 2
  spline S127 degree 2 poles (-88.1482, -5.0166) (-88.2594, -5.0487) (-88.4422, -5.0808) (-88.5805, -5.0808) knots 0 0 0 1 2 2 2
  spline S128 degree 2 poles (-88.1334, -3.6309) (-88.1383, -3.4753) (-88.2026, -3.2481) (-88.2643, -3.1715) knots 0 0 0 1 2 2 2
  spline S129 degree 2 poles (-88.2643, -3.1715) (-88.331, -3.085) (-88.541, -2.9937) (-88.6966, -2.9937) knots 0 0 0 1 2 2 2
  spline S130 degree 2 poles (-88.6966, -2.9937) (-88.8497, -2.9937) (-89.0646, -3.085) (-89.1535, -3.174) knots 0 0 0 1 2 2 2
  spline S131 degree 2 poles (-89.1535, -3.174) (-89.24, -3.2654) (-89.3289, -3.4852) (-89.3412, -3.6309) knots 0 0 0 1 2 2 2
  line L122 (-89.3412, -3.6309) -> (-88.1334, -3.6309)
  line L123 (-83.8158, -5.029) -> (-84.2209, -5.029)
  line L124 (-84.2209, -5.029) -> (-84.2209, -3.5371)
  line L125 (-84.2209, -3.5371) -> (-85.6239, -3.5371)
  line L126 (-85.6239, -3.5371) -> (-85.6239, -5.029)
  line L127 (-85.6239, -5.029) -> (-86.029, -5.029)
  line L128 (-86.029, -5.029) -> (-86.029, -1.981)
  line L129 (-86.029, -1.981) -> (-85.6239, -1.981)
  line L130 (-85.6239, -1.981) -> (-85.6239, -3.1764)
  line L131 (-85.6239, -3.1764) -> (-84.2209, -3.1764)
  line L132 (-84.2209, -3.1764) -> (-84.2209, -1.981)
  line L133 (-84.2209, -1.981) -> (-83.8158, -1.981)
  line L134 (-83.8158, -1.981) -> (-83.8158, -5.029)
  spline S132 degree 2 poles (-82.235, -5.0808) (-82.7834, -5.0808) (-83.386, -4.4658) (-83.386, -3.8977) knots 0 0 0 1 2 2 2
  spline S133 degree 2 poles (-83.386, -3.8977) (-83.386, -3.3395) (-82.8006, -2.6775) (-82.3289, -2.6775) knots 0 0 0 1 2 2 2
  spline S134 degree 2 poles (-82.3289, -2.6775) (-82.1164, -2.6775) (-81.7879, -2.801) (-81.6669, -2.9319) knots 0 0 0 1 2 2 2
  spline S135 degree 2 poles (-81.6669, -2.9319) (-81.5434, -3.0628) (-81.4125, -3.4407) (-81.4125, -3.7149) knots 0 0 0 1 2 2 2
  line L135 (-81.4125, -3.7149) -> (-81.4125, -3.9249)
  line L136 (-81.4125, -3.9249) -> (-82.9958, -3.9249)
  spline S136 degree 2 poles (-82.9958, -3.9249) (-82.9958, -4.3225) (-82.5956, -4.7449) (-82.2399, -4.7449) knots 0 0 0 1 2 2 2
  spline S137 degree 2 poles (-82.2399, -4.7449) (-82.114, -4.7449) (-81.8694, -4.6881) (-81.7706, -4.6436) knots 0 0 0 1 2 2 2
  spline S138 degree 2 poles (-81.7706, -4.6436) (-81.6669, -4.5942) (-81.5236, -4.5078) (-81.4767, -4.4683) knots 0 0 0 1 2 2 2
  line L137 (-81.4767, -4.4683) -> (-81.4545, -4.4683)
  line L138 (-81.4545, -4.4683) -> (-81.4545, -4.8882)
  spline S139 degree 2 poles (-81.4545, -4.8882) (-81.5212, -4.9153) (-81.7237, -4.9944) (-81.8028, -5.0166) knots 0 0 0 1 2 2 2
  spline S140 degree 2 poles (-81.8028, -5.0166) (-81.9139, -5.0487) (-82.0967, -5.0808) (-82.235, -5.0808) knots 0 0 0 1 2 2 2
  spline S141 degree 2 poles (-81.7879, -3.6309) (-81.7929, -3.4753) (-81.8571, -3.2481) (-81.9188, -3.1715) knots 0 0 0 1 2 2 2
  spline S142 degree 2 poles (-81.9188, -3.1715) (-81.9855, -3.085) (-82.1955, -2.9937) (-82.3511, -2.9937) knots 0 0 0 1 2 2 2
  spline S143 degree 2 poles (-82.3511, -2.9937) (-82.5042, -2.9937) (-82.7191, -3.085) (-82.8081, -3.174) knots 0 0 0 1 2 2 2
  spline S144 degree 2 poles (-82.8081, -3.174) (-82.8945, -3.2654) (-82.9834, -3.4852) (-82.9958, -3.6309) knots 0 0 0 1 2 2 2
  line L139 (-82.9958, -3.6309) -> (-81.7879, -3.6309)
  line L140 (-79.8095, -3.1542) -> (-79.8292, -3.1542)
  spline S145 degree 2 poles (-79.8292, -3.1542) (-79.8737, -3.1419) (-79.97, -3.1369) (-80.0367, -3.1369) knots 0 0 0 1 2 2 2
  spline S146 degree 2 poles (-80.0367, -3.1369) (-80.1923, -3.1369) (-80.4986, -3.2728) (-80.6369, -3.4062) knots 0 0 0 1 2 2 2
  line L141 (-80.6369, -3.4062) -> (-80.6369, -5.029)
  line L142 (-80.6369, -5.029) -> (-81.0222, -5.029)
  line L143 (-81.0222, -5.029) -> (-81.0222, -2.7417)
  line L144 (-81.0222, -2.7417) -> (-80.6369, -2.7417)
  line L145 (-80.6369, -2.7417) -> (-80.6369, -3.0826)
  spline S147 degree 2 poles (-80.6369, -3.0826) (-80.427, -2.8949) (-80.1133, -2.7417) (-79.9651, -2.7417) knots 0 0 0 1 2 2 2
  spline S148 degree 2 poles (-79.9651, -2.7417) (-79.9058, -2.7417) (-79.8465, -2.7467) (-79.8095, -2.7541) knots 0 0 0 1 2 2 2
  line L146 (-79.8095, -2.7541) -> (-79.8095, -3.1542)
  spline S149 degree 2 poles (-77.6309, -3.8853) (-77.6309, -4.4633) (-78.1867, -5.0932) (-78.651, -5.0932) knots 0 0 0 1 2 2 2
  spline S150 degree 2 poles (-78.651, -5.0932) (-79.1277, -5.0932) (-79.6736, -4.4436) (-79.6736, -3.8853) knots 0 0 0 1 2 2 2
  spline S151 degree 2 poles (-79.6736, -3.8853) (-79.6736, -3.3123) (-79.1104, -2.6775) (-78.651, -2.6775) knots 0 0 0 1 2 2 2
  spline S152 degree 2 poles (-78.651, -2.6775) (-78.1867, -2.6775) (-77.6309, -3.3098) (-77.6309, -3.8853) knots 0 0 0 1 2 2 2
  spline S153 degree 2 poles (-78.0286, -3.8853) (-78.0286, -3.4407) (-78.3521, -3.0085) (-78.651, -3.0085) knots 0 0 0 1 2 2 2
  spline S154 degree 2 poles (-78.651, -3.0085) (-78.9499, -3.0085) (-79.2759, -3.4407) (-79.2759, -3.8853) knots 0 0 0 1 2 2 2
  spline S155 degree 2 poles (-79.2759, -3.8853) (-79.2759, -4.3176) (-78.9499, -4.7622) (-78.651, -4.7622) knots 0 0 0 1 2 2 2
  spline S156 degree 2 poles (-78.651, -4.7622) (-78.3546, -4.7622) (-78.0286, -4.325) (-78.0286, -3.8853) knots 0 0 0 1 2 2 2
  line L147 (-76.843, -5.029) -> (-77.2283, -5.029)
  line L148 (-77.2283, -5.029) -> (-77.2283, -1.8451)
  line L149 (-77.2283, -1.8451) -> (-76.843, -1.8451)
  line L150 (-76.843, -1.8451) -> (-76.843, -5.029)
  line L151 (-74.5187, -5.029) -> (-74.904, -5.029)
  line L152 (-74.904, -5.029) -> (-74.904, -4.7968)
  spline S157 degree 2 poles (-74.904, -4.7968) (-74.9929, -4.8709) (-75.1238, -4.9697) (-75.2128, -5.0117) knots 0 0 0 1 2 2 2
  spline S158 degree 2 poles (-75.2128, -5.0117) (-75.2943, -5.0512) (-75.4696, -5.0932) (-75.5857, -5.0932) knots 0 0 0 1 2 2 2
  spline S159 degree 2 poles (-75.5857, -5.0932) (-75.7734, -5.0932) (-76.0896, -4.9376) (-76.2008, -4.7869) knots 0 0 0 1 2 2 2
  spline S160 degree 2 poles (-76.2008, -4.7869) (-76.3119, -4.6362) (-76.4354, -4.1916) (-76.4354, -3.9026) knots 0 0 0 1 2 2 2
  spline S161 degree 2 poles (-76.4354, -3.9026) (-76.4354, -3.6013) (-76.2798, -3.1616) (-76.1439, -2.9961) knots 0 0 0 1 2 2 2
  spline S162 degree 2 poles (-76.1439, -2.9961) (-76.018, -2.8479) (-75.6648, -2.6775) (-75.4696, -2.6775) knots 0 0 0 1 2 2 2
  spline S163 degree 2 poles (-75.4696, -2.6775) (-75.2992, -2.6775) (-75.0448, -2.7541) (-74.904, -2.8331) knots 0 0 0 1 2 2 2
  line L153 (-74.904, -2.8331) -> (-74.904, -1.8451)
  line L154 (-74.904, -1.8451) -> (-74.5187, -1.8451)
  line L155 (-74.5187, -1.8451) -> (-74.5187, -5.029)
  line L156 (-74.904, -4.4732) -> (-74.904, -3.1517)
  spline S164 degree 2 poles (-74.904, -3.1517) (-75.0473, -3.0826) (-75.2745, -3.0307) (-75.4054, -3.0307) knots 0 0 0 1 2 2 2
  spline S165 degree 2 poles (-75.4054, -3.0307) (-75.7018, -3.0307) (-76.0377, -3.4753) (-76.0377, -3.8952) knots 0 0 0 1 2 2 2
  spline S166 degree 2 poles (-76.0377, -3.8952) (-76.0377, -4.3003) (-75.7809, -4.7276) (-75.4968, -4.7276) knots 0 0 0 1 2 2 2
  spline S167 degree 2 poles (-75.4968, -4.7276) (-75.3461, -4.7276) (-75.0399, -4.5893) (-74.904, -4.4732) knots 0 0 0 1 2 2 2
  line L157 (-71.5917, -3.8804) -> (-72.7452, -3.8804)
  line L158 (-72.7452, -3.8804) -> (-72.7452, -3.5099)
  line L159 (-72.7452, -3.5099) -> (-71.5917, -3.5099)
  line L160 (-71.5917, -3.5099) -> (-71.5917, -3.8804)
  spline S168 degree 2 poles (-67.7237, -4.0928) (-67.7237, -4.3201) (-67.8966, -4.6683) (-68.0398, -4.782) knots 0 0 0 1 2 2 2
  spline S169 degree 2 poles (-68.0398, -4.782) (-68.2127, -4.9153) (-68.6055, -5.029) (-68.9167, -5.029) knots 0 0 0 1 2 2 2
  line L161 (-68.9167, -5.029) -> (-69.7911, -5.029)
  line L162 (-69.7911, -5.029) -> (-69.7911, -1.981)
  line L163 (-69.7911, -1.981) -> (-68.9834, -1.981)
  spline S170 degree 2 poles (-68.9834, -1.981) (-68.6573, -1.981) (-68.3313, -2.0229) (-68.1831, -2.1045) knots 0 0 0 1 2 2 2
  spline S171 degree 2 poles (-68.1831, -2.1045) (-68.0176, -2.1909) (-67.8669, -2.475) (-67.8669, -2.6676) knots 0 0 0 1 2 2 2
  spline S172 degree 2 poles (-67.8669, -2.6676) (-67.8669, -2.8825) (-68.0942, -3.2234) (-68.2942, -3.3197) knots 0 0 0 1 2 2 2
  line L164 (-68.2942, -3.3197) -> (-68.2942, -3.3345)
  spline S173 degree 2 poles (-68.2942, -3.3345) (-68.0225, -3.4086) (-67.7237, -3.8014) (-67.7237, -4.0928) knots 0 0 0 1 2 2 2
  spline S174 degree 2 poles (-68.146, -4.1101) (-68.146, -3.9372) (-68.2448, -3.7149) (-68.393, -3.6359) knots 0 0 0 1 2 2 2
  spline S175 degree 2 poles (-68.393, -3.6359) (-68.4894, -3.5865) (-68.7166, -3.5568) (-68.9266, -3.5568) knots 0 0 0 1 2 2 2
  line L165 (-68.9266, -3.5568) -> (-69.386, -3.5568)
  line L166 (-69.386, -3.5568) -> (-69.386, -4.6831)
  line L167 (-69.386, -4.6831) -> (-69.0575, -4.6831)
  spline S176 degree 2 poles (-69.0575, -4.6831) (-68.7907, -4.6831) (-68.4844, -4.6337) (-68.3659, -4.5547) knots 0 0 0 1 2 2 2
  spline S177 degree 2 poles (-68.3659, -4.5547) (-68.2522, -4.4732) (-68.146, -4.2707) (-68.146, -4.1101) knots 0 0 0 1 2 2 2
  spline S178 degree 2 poles (-68.2893, -2.7244) (-68.2893, -2.6157) (-68.3634, -2.4527) (-68.4449, -2.4058) knots 0 0 0 1 2 2 2
  spline S179 degree 2 poles (-68.4449, -2.4058) (-68.5437, -2.3515) (-68.7833, -2.3268) (-68.9982, -2.3268) knots 0 0 0 1 2 2 2
  line L168 (-68.9982, -2.3268) -> (-69.386, -2.3268)
  line L169 (-69.386, -2.3268) -> (-69.386, -3.2184)
  line L170 (-69.386, -3.2184) -> (-68.9266, -3.2184)
  spline S180 degree 2 poles (-68.9266, -3.2184) (-68.7364, -3.2184) (-68.5561, -3.1789) (-68.4597, -3.1172) knots 0 0 0 1 2 2 2
  spline S181 degree 2 poles (-68.4597, -3.1172) (-68.3659, -3.0579) (-68.2893, -2.8677) (-68.2893, -2.7244) knots 0 0 0 1 2 2 2
  line L171 (-66.1379, -3.1542) -> (-66.1577, -3.1542)
  spline S182 degree 2 poles (-66.1577, -3.1542) (-66.2021, -3.1419) (-66.2985, -3.1369) (-66.3652, -3.1369) knots 0 0 0 1 2 2 2
  spline S183 degree 2 poles (-66.3652, -3.1369) (-66.5208, -3.1369) (-66.827, -3.2728) (-66.9654, -3.4062) knots 0 0 0 1 2 2 2
  line L172 (-66.9654, -3.4062) -> (-66.9654, -5.029)
  line L173 (-66.9654, -5.029) -> (-67.3507, -5.029)
  line L174 (-67.3507, -5.029) -> (-67.3507, -2.7417)
  line L175 (-67.3507, -2.7417) -> (-66.9654, -2.7417)
  line L176 (-66.9654, -2.7417) -> (-66.9654, -3.0826)
  spline S184 degree 2 poles (-66.9654, -3.0826) (-66.7554, -2.8949) (-66.4417, -2.7417) (-66.2935, -2.7417) knots 0 0 0 1 2 2 2
  spline S185 degree 2 poles (-66.2935, -2.7417) (-66.2342, -2.7417) (-66.175, -2.7467) (-66.1379, -2.7541) knots 0 0 0 1 2 2 2
  line L177 (-66.1379, -2.7541) -> (-66.1379, -3.1542)
  spline S186 degree 2 poles (-63.9594, -3.8853) (-63.9594, -4.4633) (-64.5151, -5.0932) (-64.9795, -5.0932) knots 0 0 0 1 2 2 2
  spline S187 degree 2 poles (-64.9795, -5.0932) (-65.4562, -5.0932) (-66.0021, -4.4436) (-66.0021, -3.8853) knots 0 0 0 1 2 2 2
  spline S188 degree 2 poles (-66.0021, -3.8853) (-66.0021, -3.3123) (-65.4389, -2.6775) (-64.9795, -2.6775) knots 0 0 0 1 2 2 2
  spline S189 degree 2 poles (-64.9795, -2.6775) (-64.5151, -2.6775) (-63.9594, -3.3098) (-63.9594, -3.8853) knots 0 0 0 1 2 2 2
  spline S190 degree 2 poles (-64.357, -3.8853) (-64.357, -3.4407) (-64.6806, -3.0085) (-64.9795, -3.0085) knots 0 0 0 1 2 2 2
  spline S191 degree 2 poles (-64.9795, -3.0085) (-65.2783, -3.0085) (-65.6044, -3.4407) (-65.6044, -3.8853) knots 0 0 0 1 2 2 2
  spline S192 degree 2 poles (-65.6044, -3.8853) (-65.6044, -4.3176) (-65.2783, -4.7622) (-64.9795, -4.7622) knots 0 0 0 1 2 2 2
  spline S193 degree 2 poles (-64.9795, -4.7622) (-64.6831, -4.7622) (-64.357, -4.325) (-64.357, -3.8853) knots 0 0 0 1 2 2 2
  line L178 (-61.8055, -5.029) -> (-62.1908, -5.029)
  line L179 (-62.1908, -5.029) -> (-62.1908, -4.7968)
  spline S194 degree 2 poles (-62.1908, -4.7968) (-62.2797, -4.8709) (-62.4107, -4.9697) (-62.4996, -5.0117) knots 0 0 0 1 2 2 2
  spline S195 degree 2 poles (-62.4996, -5.0117) (-62.5811, -5.0512) (-62.7565, -5.0932) (-62.8726, -5.0932) knots 0 0 0 1 2 2 2
  spline S196 degree 2 poles (-62.8726, -5.0932) (-63.0603, -5.0932) (-63.3764, -4.9376) (-63.4876, -4.7869) knots 0 0 0 1 2 2 2
  spline S197 degree 2 poles (-63.4876, -4.7869) (-63.5987, -4.6362) (-63.7222, -4.1916) (-63.7222, -3.9026) knots 0 0 0 1 2 2 2
  spline S198 degree 2 poles (-63.7222, -3.9026) (-63.7222, -3.6013) (-63.5666, -3.1616) (-63.4308, -2.9961) knots 0 0 0 1 2 2 2
  spline S199 degree 2 poles (-63.4308, -2.9961) (-63.3048, -2.8479) (-62.9516, -2.6775) (-62.7565, -2.6775) knots 0 0 0 1 2 2 2
  spline S200 degree 2 poles (-62.7565, -2.6775) (-62.586, -2.6775) (-62.3316, -2.7541) (-62.1908, -2.8331) knots 0 0 0 1 2 2 2
  line L180 (-62.1908, -2.8331) -> (-62.1908, -1.8451)
  line L181 (-62.1908, -1.8451) -> (-61.8055, -1.8451)
  line L182 (-61.8055, -1.8451) -> (-61.8055, -5.029)
  line L183 (-62.1908, -4.4732) -> (-62.1908, -3.1517)
  spline S201 degree 2 poles (-62.1908, -3.1517) (-62.3341, -3.0826) (-62.5613, -3.0307) (-62.6922, -3.0307) knots 0 0 0 1 2 2 2
  spline S202 degree 2 poles (-62.6922, -3.0307) (-62.9886, -3.0307) (-63.3246, -3.4753) (-63.3246, -3.8952) knots 0 0 0 1 2 2 2
  spline S203 degree 2 poles (-63.3246, -3.8952) (-63.3246, -4.3003) (-63.0677, -4.7276) (-62.7836, -4.7276) knots 0 0 0 1 2 2 2
  spline S204 degree 2 poles (-62.7836, -4.7276) (-62.633, -4.7276) (-62.3267, -4.5893) (-62.1908, -4.4732) knots 0 0 0 1 2 2 2
  line L184 (-60.8545, -5.029) -> (-61.2399, -5.029)
  line L185 (-61.2399, -5.029) -> (-61.2399, -2.7417)
  line L186 (-61.2399, -2.7417) -> (-60.8545, -2.7417)
  line L187 (-60.8545, -2.7417) -> (-60.8545, -5.029)
  line L188 (-60.8274, -2.3613) -> (-61.2646, -2.3613)
  line L189 (-61.2646, -2.3613) -> (-61.2646, -1.9612)
  line L190 (-61.2646, -1.9612) -> (-60.8274, -1.9612)
  line L191 (-60.8274, -1.9612) -> (-60.8274, -2.3613)
  spline S205 degree 2 poles (-59.296, -5.0808) (-59.8443, -5.0808) (-60.447, -4.4658) (-60.447, -3.8977) knots 0 0 0 1 2 2 2
  spline S206 degree 2 poles (-60.447, -3.8977) (-60.447, -3.3395) (-59.8616, -2.6775) (-59.3898, -2.6775) knots 0 0 0 1 2 2 2
  spline S207 degree 2 poles (-59.3898, -2.6775) (-59.1774, -2.6775) (-58.8489, -2.801) (-58.7279, -2.9319) knots 0 0 0 1 2 2 2
  spline S208 degree 2 poles (-58.7279, -2.9319) (-58.6044, -3.0628) (-58.4735, -3.4407) (-58.4735, -3.7149) knots 0 0 0 1 2 2 2
  line L192 (-58.4735, -3.7149) -> (-58.4735, -3.9249)
  line L193 (-58.4735, -3.9249) -> (-60.0567, -3.9249)
  spline S209 degree 2 poles (-60.0567, -3.9249) (-60.0567, -4.3225) (-59.6566, -4.7449) (-59.3009, -4.7449) knots 0 0 0 1 2 2 2
  spline S210 degree 2 poles (-59.3009, -4.7449) (-59.1749, -4.7449) (-58.9304, -4.6881) (-58.8316, -4.6436) knots 0 0 0 1 2 2 2
  spline S211 degree 2 poles (-58.8316, -4.6436) (-58.7279, -4.5942) (-58.5846, -4.5078) (-58.5377, -4.4683) knots 0 0 0 1 2 2 2
  line L194 (-58.5377, -4.4683) -> (-58.5154, -4.4683)
  line L195 (-58.5154, -4.4683) -> (-58.5154, -4.8882)
  spline S212 degree 2 poles (-58.5154, -4.8882) (-58.5821, -4.9153) (-58.7847, -4.9944) (-58.8637, -5.0166) knots 0 0 0 1 2 2 2
  spline S213 degree 2 poles (-58.8637, -5.0166) (-58.9749, -5.0487) (-59.1576, -5.0808) (-59.296, -5.0808) knots 0 0 0 1 2 2 2
  spline S214 degree 2 poles (-58.8489, -3.6309) (-58.8538, -3.4753) (-58.9181, -3.2481) (-58.9798, -3.1715) knots 0 0 0 1 2 2 2
  spline S215 degree 2 poles (-58.9798, -3.1715) (-59.0465, -3.085) (-59.2564, -2.9937) (-59.4121, -2.9937) knots 0 0 0 1 2 2 2
  spline S216 degree 2 poles (-59.4121, -2.9937) (-59.5652, -2.9937) (-59.7801, -3.085) (-59.869, -3.174) knots 0 0 0 1 2 2 2